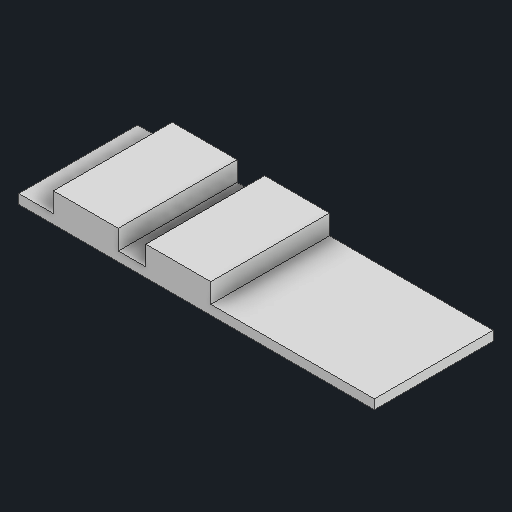
# Autodesk Inventor part: BMS
Saved by Autodesk Inventor 2027.1 (Build 311270010, 270A)
## iProperties
Created: 2026-08-07
Part Number: BMS
Material: 일반
Document SubType Name: Modeling
Designer: moieboy9999
Density: 2.08059 g/cm^3
Appearance: 기본값
Mass: 3 g
Surface Area: 17.4326 cm^2
Volume: 1.4419 cm^3
Author: moieboy9999
Autodesk Inventor part; units mm, degrees
ref_plane "YZ Plane" through (0, 0, 0) normal (1, 0, 0) x (0, 1, 0)
ref_plane "XZ Plane" through (0, 0, 0) normal (0, 1, 0) x (-1, 0, 0)
ref_plane "XY Plane" through (0, 0, 0) normal (0, 0, 1) x (1, 0, 0)
sketch "스케치1" plane through (0, 0, 0) normal (0, 1, 0) x (-1, 0, 0)
  line L0 (0, 0) -> (-45.2, 0)
  line L1 (-45.2, 0) -> (-45.2, -15.1)
  line L2 (-45.2, -15.1) -> (0, -15.1)
  line L3 (0, -15.1) -> (0, 0)
  dimension "d0" = 45.2
  dimension "d1" = 15.1
  constraints: 8 end point, 2 parallel, 1 horizontal, 1 perpendicular
  measures "d0" distance of L2.end L1.end
  measures "d1" distance of L1.end L0.end
extrude "돌출1" add sketch "스케치1" along normal blind 3.7
sketch "스케치2" plane through (0, 3.7, 0) normal (0, 1, 0) x (1, 0, 0)
  line L0 (0, 0) -> (45.2, 0) projected
  line L1 (45.2, 15.1) -> (0, 15.1) projected
  line L2 (0, 0) -> (4.4, 0)
  line L3 (4.4, 0) -> (4.4, 15.1)
  line L4 (4.4, 15.1) -> (0, 15.1)
  line L5 (0, 15.1) -> (0, 0)
  line L6 (4.4, 15.1) -> (14.4, 15.1)
  line L7 (14.4, 15.1) -> (14.4, 0)
  line L8 (14.4, 0) -> (4.4, 0)
  line L9 (4.4, 0) -> (4.4, 15.1)
  line L10 (14.4, 0) -> (13.4, 0)
  line L11 (13.4, 0) -> (15.4, 0)
  line L12 (13.4, 0) -> (5.6, 0)
  line L13 (5.6, 0) -> (5.6, 15.1)
  line L14 (5.6, 15.1) -> (13.4, 15.1)
  line L15 (13.4, 15.1) -> (13.4, 0)
  line L16 (15.4, 0) -> (23.2, 0)
  line L17 (23.2, 0) -> (23.2, 15.1)
  line L18 (23.2, 15.1) -> (15.4, 15.1)
  line L19 (15.4, 15.1) -> (15.4, 0)
  line L20 (23.2, 15.1) -> (45.2, 15.1)
  line L21 (45.2, 15.1) -> (45.2, 0)
  line L22 (45.2, 0) -> (23.2, 0)
  line L23 (23.2, 0) -> (23.2, 15.1)
  dimension "d4" = 4.4
  dimension "d5" = 10
  dimension "d6" = 1
  dimension "d7" = 2
  dimension "d8" = 7.8
  dimension "d9" = 7.8
  constraints: 44 end point, 10 parallel, 6 point on line, 5 horizontal, 5 perpendicular
  measures "d4" distance of L4.end L3.end
  measures "d5" distance of L7.end L8.end
  measures "d6" distance of L7.end L10.end
  measures "d7" distance of L10.end L11.end
  measures "d8" distance of L13.end L14.end
  measures "d9" distance of L18.end L17.end
extrude "돌출2" cut sketch "스케치2" against normal blind 2.5 contours L5 L1 L3 L0 | L15 L1 L7 L0 | L7 L1 L19 L0 | L17 L1 L21 L0
offset faces "크기1" outward -0.75 faces at (13.4, 2.8667, -10.0667) (15.4, 2.8667, -5.0333)
offset faces "크기2" outward 1.2 faces at (23.2, 2.0333, -5.0333)
